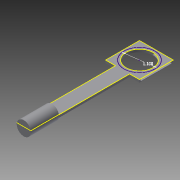
# Autodesk Inventor part: Silicon Frame v2
Saved by Autodesk Inventor 2014 SP2 (Build 180246200, 246)
## iProperties
Created: 2014-10-11
Part Number: Silicon Frame v2
Material: Generic
Document SubType Name: Modeling
Designer: Henry Bishop
Density: 1 g/cm^3
Appearance: Default
Author: Henry Bishop
Autodesk Inventor part; units mm, degrees
ref_plane "YZ Plane" through (0, 0, 0) normal (1, 0, 0) x (0, 1, 0)
ref_plane "XZ Plane" through (0, 0, 0) normal (0, 1, 0) x (-1, 0, 0)
ref_plane "XY Plane" through (0, 0, 0) normal (0, 0, 1) x (1, 0, 0)
sketch "Sketch1" plane through (0, 0, 0) normal (0, 1, 0) x (-1, 0, 0)
  line L0 (15.24, -15.24) -> (-15.24, -15.24)
  line L1 (-15.24, -15.24) -> (-15.24, 15.24)
  line L2 (-15.24, 15.24) -> (15.24, 15.24)
  line L3 (15.24, 15.24) -> (15.24, -15.24)
  line L4 (15.24, -15.24) -> (-15.24, 15.24) construction
  line L5 (-15.24, -15.24) -> (15.24, 15.24) construction
  circle A0 centre (0, 0) radius 15.24
  dimension "d0" = 30.48
  dimension "d3" = 30.48
  constraints: 12 end point, 2 midpoint, 2 parallel, 1 centre point, 1 coincident, 1 horizontal, 1 perpendicular
  measures "d0" distance of L1.end L2.end
  measures "d3" distance of L0.start L2.end
extrude "Extrusion1" add sketch "Sketch1" along normal blind 2.54
sketch "Sketch2" plane through (-15.24, 0, 15.24) normal (0, 0, 1) x (1, 0, 0)
  line L0 (30.48, 0) -> (0, 0) projected
  line L1 (8.8466, 2.54) -> (21.6334, 2.54)
  line L2 (21.6334, 2.54) -> (21.6334, 0)
  line L3 (21.6334, 0) -> (8.8466, 0)
  line L4 (8.8466, 0) -> (8.8466, 2.54)
  line L5 (8.8466, 2.54) -> (21.6334, 0) construction
  line L6 (21.6334, 2.54) -> (8.8466, 0) construction
  point P0 (15.24, 0)
  point P1 (15.24, 1.27)
  constraints: 12 end point, 2 midpoint, 2 parallel, 1 horizontal, 1 perpendicular, 1 point on line
extrude "Extrusion2" add sketch "Sketch2" along normal blind 63.5
sketch "Sketch5" plane through (-15.24, 0, 78.74) normal (0, 0, 1) x (1, 0, 0)
  circle A0 centre (15.24, 1.27) radius 6.35
  point P0 (15.24, 0)
  dimension "d14" = 12.7
  constraints: 1 centre point
  measures "d14" diameter of A0
extrude "Extrusion5" add sketch "Sketch5" along normal blind 25.4
sketch "Sketch7" plane through (15.24, 0, 15.24) normal (1, 0, 0) x (0, 0, -1)
  line L0 (1.27, 2.032) -> (29.21, 2.032)
  line L1 (29.21, 2.032) -> (29.21, 0.508)
  line L2 (29.21, 0.508) -> (1.27, 0.508)
  line L3 (1.27, 0.508) -> (1.27, 2.032)
  line L4 (1.27, 2.032) -> (29.21, 0.508) construction
  line L5 (29.21, 2.032) -> (1.27, 0.508) construction
  point P0 (15.24, 0)
  point P1 (15.24, 1.27)
  dimension "d35" = 27.94
  dimension "d36" = 1.524
  constraints: 12 end point, 2 midpoint, 2 parallel, 1 horizontal, 1 perpendicular
  measures "d35" distance of L1.end L2.end
  measures "d36" distance of L0.end L1.end
extrude "Extrusion7" cut sketch "Sketch7" against normal blind 15.24
sketch "Sketch8" plane through (0, 2.54, 0) normal (0, 1, 0) x (1, 0, 0)
  circle A0 centre (0, 0) radius 12.065
  dimension "d39" = 24.13
  constraints: 1 centre point, 1 coincident
  measures "d39" diameter of A0
extrude "Extrusion8" cut sketch "Sketch8" against normal blind 31.75
sketch "Sketch9" plane through (0, 2.54, 0) normal (0, 1, 0) x (1, 0, 0)
  circle A0 centre (0, 0) radius 12.065 projected
  line L0 (15.24, 15.24) -> (-15.24, 15.24) projected
  line L1 (-15.24, 15.24) -> (-15.24, -15.24) projected
  line L2 (-15.24, -15.24) -> (-6.3934, -15.24) projected
  line L3 (-6.3934, -15.24) -> (-6.3934, -78.74) projected
  line L4 (-6.2217, -78.74) -> (-6.3934, -78.74) projected
  line L5 (6.2217, -78.74) -> (-6.2217, -78.74) projected
  line L6 (6.3934, -78.74) -> (6.2217, -78.74) projected
  line L7 (6.3934, -15.24) -> (6.3934, -78.74) projected
  line L8 (6.3934, -15.24) -> (15.24, -15.24) projected
  line L9 (15.24, -15.24) -> (15.24, 15.24) projected
  circle A1 centre (0, 0) radius 13.97
  circle A2 centre (0, 0) radius 12.065 projected
  line L10 (-6.2217, -78.74) -> (6.2217, -78.74) projected
  line L11 (6.2217, -78.74) -> (6.2217, -104.14) projected
  line L12 (6.2217, -104.14) -> (-6.2217, -104.14) projected
  line L13 (-6.2217, -104.14) -> (-6.2217, -78.74) projected
  line L14 (-6.2217, -78.74) -> (-6.3934, -78.74) projected
  line L15 (-6.3934, -78.74) -> (-6.3934, -15.24) projected
  line L16 (-6.3934, -15.24) -> (-15.24, -15.24) projected
  line L17 (-15.24, -15.24) -> (-15.24, 15.24) projected
  line L18 (-15.24, 15.24) -> (15.24, 15.24) projected
  line L19 (15.24, 15.24) -> (15.24, -15.24) projected
  line L20 (15.24, -15.24) -> (6.3934, -15.24) projected
  line L21 (6.3934, -15.24) -> (6.3934, -78.74) projected
  line L22 (6.3934, -78.74) -> (6.2217, -78.74) projected
  dimension "d42" = 27.94
  constraints: 1 centre point, 1 coincident
  measures "d42" diameter of A1
body "Solid1"
